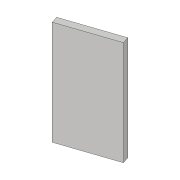
# Autodesk Inventor part: Lidar Sensor Case Piece 4
Saved by Autodesk Inventor 2018.3 (Build 223284000, 284)
## iProperties
Created: 2019-02-26
Part Number: Lidar Sensor Case Piece 4
Material: Generic
Document SubType Name: Modeling
Designer: aye06091
Mass: 4.10086 g
Surface Area: 30.6145 cm^2
Volume: 4.10086 cm^3
Density: 1 g/cm^3
Appearance: Default
Author: aye06091
Autodesk Inventor part; units mm, degrees
ref_plane "YZ Plane" through (0, 0, 0) normal (1, 0, 0) x (0, 1, 0)
ref_plane "XZ Plane" through (0, 0, 0) normal (0, 1, 0) x (-1, 0, 0)
ref_plane "XY Plane" through (0, 0, 0) normal (0, 0, 1) x (1, 0, 0)
sketch "Sketch1" plane through (0, 0, 0) normal (0, 1, 0) x (-1, 0, 0)
  line L0 (-2.011, 9.1787) -> (-27.0562, 0.7795)
  line L1 (-28.0657, 3.7897) -> (-3.0206, 12.189)
  line L2 (-2.011, 9.1787) -> (-3.0206, 12.189)
  line L3 (-27.0562, 0.7795) -> (-28.0657, 3.7897)
  point P0 (0, 0)
  point P1 (-9.862, 5.3709)
  dimension "d0" = 26.416
  constraints: 8 end point
  measures "d0" distance of L0.start L0.end
extrude "Extrusion1" add sketch "Sketch1" along normal blind 48.895
body "Solid1"
